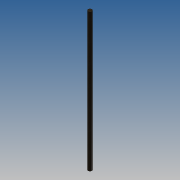
# Autodesk Inventor part: 2p2pol
Saved by Autodesk Inventor 2014 SP1 (Build 180222100, 222)
## iProperties
Company: HERA Project
Created: 2013-05-22
Part Number: 2p2pol
Material: Wood (Maple)
Document SubType Name: Modeling
Designer: David DeBoer
Density: 0.57 g/cm^3
Description: support pole
Mass: 110908 g
Surface Area: 38950.9 cm^2
Volume: 194576 cm^3
Appearance: Natural Maple - Glossy Dark Tint
Author: David DeBoer
Title: Support pole
Autodesk Inventor part; units mm, degrees
ref_plane "YZ Plane" through (0, 0, 0) normal (1, 0, 0) x (0, 1, 0)
ref_plane "XZ Plane" through (0, 0, 0) normal (0, 1, 0) x (-1, 0, 0)
ref_plane "XY Plane" through (0, 0, 0) normal (0, 0, 1) x (1, 0, 0)
sketch "Sketch1" plane through (0, 0, 0) normal (0, 1, 0) x (-1, 0, 0)
  circle A0 centre (0, 0) radius 101.6
  dimension "d0" = 203.2
  constraints: 1 centre point, 1 coincident
  measures "d0" diameter of A0
extrude "Extrusion1" add sketch "Sketch1" along normal blind 7000
sketch "Sketch2" plane through (0, 0, 0) normal (0, -1, 0) x (1, 0, 0)
  circle A0 centre (0, 0) radius 101.6 projected
extrude "Extrusion2" [suppressed]
sketch "Sketch3" plane through (0, 7000, 0) normal (0, 1, 0) x (1, 0, 0)
  circle A0 centre (0, 0) radius 101.6 projected
  point P0 (101.6, 0)
  constraints: 1 horizontal alignment, 1 other
ref_plane "Work Plane1" through (101.6, 7000, 0) normal (1, 0, 0) x (0, 1, 0)
sketch "Sketch4" plane through (101.6, 7000, 0) normal (1, 0, 0) x (0, 1, 0)
  line L0 (-3724.2493, -34.0955) -> (-3560.2966, -34.0955)
  line L1 (-3560.2966, -34.0955) -> (-3560.2966, 34.0407)
  line L2 (-3560.2966, 34.0407) -> (-3724.2493, 34.0407)
  line L3 (-3724.2493, 34.0407) -> (-3724.2493, -34.0955)
  line L4 (-3724.2493, -0.0274) -> (-3560.2966, -0.0274) construction
  point P0 (-7000, 0)
  constraints: 10 end point, 2 midpoint, 2 parallel, 1 horizontal, 1 perpendicular
extrude "poleStandRadialRef" cut sketch "Sketch4" against normal blind 0.254
sketch "Sketch5" plane through (0, 7000, 0) normal (0, 1, 0) x (1, 0, 0)
  circle A0 centre (0, 0) radius 101.6 projected
  point P0 (0, 101.6)
  constraints: 1 vertical alignment, 1 other
ref_plane "Work Plane2" through (0, 7000, -101.6) normal (0, 0, -1) x (-1, 0, 0)
sketch "Sketch6" plane through (0, 7000, -101.6) normal (0, 0, -1) x (-1, 0, 0)
  line L0 (-25.3983, -3556.136) -> (25.4017, -3556.136)
  line L1 (25.4017, -3556.136) -> (25.4017, -3632.336)
  line L2 (25.4017, -3632.336) -> (-25.3983, -3632.336)
  line L3 (-25.3983, -3632.336) -> (-25.3983, -3556.136)
  line L4 (0.0017, -3556.136) -> (0.0017, -3632.336) construction
  point P0 (0, -7000)
  dimension "d7" = 50.8
  dimension "d8" = 76.2
  constraints: 10 end point, 2 midpoint, 2 parallel, 1 horizontal, 1 perpendicular
  measures "d7" distance of L1.end L2.end
  measures "d8" distance of L2.end L0.start
extrude "poleStandOffsetRef" cut sketch "Sketch6" against normal blind 0.254
sketch "Sketch7" plane through (101.6, 7000, 0) normal (1, 0, 0) x (0, 1, 0)
  circle A0 centre (-304.8, 0) radius 6.35
  line L0 (0, -101.6) -> (0, 101.6) projected
  point P0 (-7000, 0)
  dimension "d11" = 12.7
  dimension "d12" = 304.8
  constraints: 1 centre point
  measures "d11" diameter of A0
  measures "d12" distance from line of A0.centre L0
extrude "eyeBoltHole" cut sketch "Sketch7" against normal blind 25.4
sketch "Sketch8" plane through (101.6, 7000, 0) normal (1, 0, 0) x (0, 1, 0)
  circle A0 centre (-4460, 0) radius 6.35
  point P0 (-7000, 0)
  dimension "d15" = 12.7
  dimension "d16" = 2540
  constraints: 1 centre point
  measures "d15" diameter of A0
  measures "d16" distance of point (-7000, 0) A0.centre
extrude "Extrusion6" cut sketch "Sketch8" against normal blind 25.4
body "Solid1"
